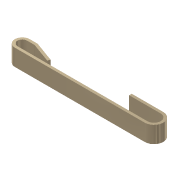
# Autodesk Inventor part: PP-13
Saved by Autodesk Inventor 2022 (Build 260148000, 148)
## iProperties
Created: 2008-09-23
Part Number: PP-13
Document SubType Name: Modeling
Designer: Mark Flayler
Mass: 1.56408 g
Surface Area: 6.64306 cm^2
Volume: 0.199245 cm^3
Density: 7.85 g/cm^3
Material: Steel
Description: CLIP
Appearance: Titanium - Polished
Author: Mark Flayler
Autodesk Inventor part; units mm, degrees
ref_plane "YZ Plane" through (0, 0, 0) normal (1, 0, 0) x (0, 1, 0)
ref_plane "XZ Plane" through (0, 0, 0) normal (0, 1, 0) x (-1, 0, 0)
ref_plane "XY Plane" through (0, 0, 0) normal (0, 0, 1) x (1, 0, 0)
sketch "Sketch1" plane through (0, 0, 0) normal (0, 0, 1) x (1, 0, 0)
  line L0 (-26.5, -5) -> (8.5, -5)
  arc A0 (8.5, -5) -> (8.5, 0) centre (8.5, -2.5) ccw
  line L1 (8.5, 0) -> (0, 0)
  arc A1 (-26.5, -1) -> (-26.5, -5) centre (-26.5, -3) ccw
  line L2 (-26.5, -1) -> (-24.63, -1)
  line L3 (-24.117, -1.0905) -> (-18.8919, -2.9922)
  arc A2 (-24.117, -1.0905) -> (-24.63, -1) centre (-24.63, -2.5) ccw
  line L4 (-18.8919, -2.9922) -> (-19.1314, -3.65) construction
  dimension "d0" = 35
  dimension "d1" = 2.5
  dimension "d2" = 8.5
  dimension "d3" = 1.5
  dimension "d5" = 20
  dimension "d6" = 1.87
  dimension "d7" = 2
  dimension "d8" = 0.7
  dimension "d9" = 1.35
  constraints: 10 end point, 6 point on circle, 6 tangent, 3 centre point, 2 parallel, 1 coincident, 1 horizontal, 1 perpendicular
  measures "d0" distance of L0.start L0.end
  measures "d1" radius of A0
  measures "d2" horizontal distance of L1.end A0.centre
  measures "d3" radius of A2
  measures "d5" angle of L0 L3
  measures "d6" distance of L2.start L2.end
  measures "d7" radius of A1
  measures "d8" distance of L3.end L4.end
  measures "d9" distance from line of L0 L4.end
sketch "Sketch2" plane through (0, 0, 0) normal (1, 0, 0) x (0, 1, 0)
  line L0 (0, 0) -> (-0.7, 0)
  line L1 (-0.7, 0) -> (-0.7, 4.5)
  line L2 (-0.7, 4.5) -> (0, 4.5)
  line L3 (0, 4.5) -> (0, 0)
  dimension "d10" = 0.7
  dimension "d11" = 4.5
  constraints: 8 end point, 2 parallel, 1 horizontal, 1 perpendicular
  measures "d10" distance of L1.end L2.end
  measures "d11" distance of L2.end L0.start
sweep "Sweep1" add profiles "Sketch2" path "Sketch1"
body "Solid1"
